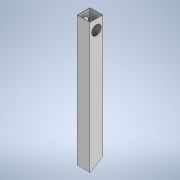
# Autodesk Inventor part: опора кинематик стенд
Saved by Autodesk Inventor 2022.4 (Build 264492010, 492A)
## iProperties
Created: 2023-02-20
Part Number: опора кинематик стенд
Material: Типовые
Document SubType Name: Modeling
Designer: artyo
Density: 1 g/cm^3
Appearance: По умолчанию
Author: artyo
Autodesk Inventor part; units mm, degrees
ref_plane "YZ Plane" through (0, 0, 0) normal (1, 0, 0) x (0, 1, 0)
ref_plane "XZ Plane" through (0, 0, 0) normal (0, 1, 0) x (-1, 0, 0)
ref_plane "XY Plane" through (0, 0, 0) normal (0, 0, 1) x (1, 0, 0)
sketch "Эскиз1" plane through (0, 0, 0) normal (0, 1, 0) x (-1, 0, 0)
  line L0 (-10, -10) -> (10, -10)
  line L1 (10, -10) -> (10, 10)
  line L2 (10, 10) -> (-10, 10)
  line L3 (-10, 10) -> (-10, -10)
  line L4 (-10, -10) -> (10, 10) construction
  line L5 (10, -10) -> (-10, 10) construction
  line L6 (-9.25, -9.25) -> (9.25, -9.25)
  line L7 (9.25, -9.25) -> (9.25, 9.25)
  line L8 (9.25, 9.25) -> (-9.25, 9.25)
  line L9 (-9.25, 9.25) -> (-9.25, -9.25)
  line L10 (-9.25, -9.25) -> (9.25, 9.25) construction
  line L11 (9.25, -9.25) -> (-9.25, 9.25) construction
  point P0 (0, 0)
  dimension "d0" = 20
  dimension "d1" = 20
  dimension "d2" = 18.5
  dimension "d3" = 18.5
  constraints: 24 end point, 4 midpoint, 4 parallel, 2 horizontal, 2 perpendicular
  measures "d0" distance of L2.end L1.end
  measures "d1" distance of L1.end L0.end
  measures "d2" distance of L8.end L7.end
  measures "d3" distance of L7.end L6.end
extrude "Выдавливание1" add sketch "Эскиз1" along normal blind 200
sketch "Эскиз2" plane through (10, 0, 10) normal (1, 0, 0) x (0, 0, -1)
  line L0 (0, 0) -> (20, 0) projected
  line L1 (0, 0) -> (20, 11.547)
  line L2 (20, 0) -> (20, 200) projected
  line L3 (0, 0) -> (23.094, 0) construction
  line L4 (0, 0) -> (20, 0)
  line L5 (19.25, 0) -> (0.75, 0) projected
  line L6 (20, 11.547) -> (20, 0)
  point P0 (10, 0)
  dimension "d6" = 30
  constraints: 8 end point, 1 collinear, 1 equal length, 1 horizontal, 1 perpendicular, 1 point on line
  measures "d6" angle of L3 L1
extrude "Выдавливание2" cut sketch "Эскиз2" against normal blind 200
sketch "Эскиз4" plane through (10, 200, 10) normal (1, 0, 0) x (0, 0, -1)
  circle A0 centre (10, -15.1881) radius 7.5
  point P0 (10, -200)
  dimension "d9" = 15
  constraints: 1 centre point
  measures "d9" diameter of A0
extrude "Выдавливание3" cut sketch "Эскиз4" against normal blind 124
